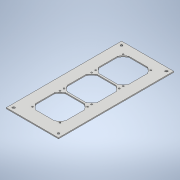
# Autodesk Inventor part: front_panel2
Saved by Autodesk Inventor 2022 (Build 260153000, 153)
## iProperties
Created: 2021-05-14
Part Number: front_panel2
Material: Generic
Document SubType Name: Modeling
Designer: gisen
Density: 1 g/cm^3
Appearance: Default
Author: gisen
Autodesk Inventor part; units mm, degrees
ref_plane "YZ Plane" through (0, 0, 0) normal (1, 0, 0) x (0, 1, 0)
ref_plane "XZ Plane" through (0, 0, 0) normal (0, 1, 0) x (-1, 0, 0)
ref_plane "XY Plane" through (0, 0, 0) normal (0, 0, 1) x (1, 0, 0)
sketch "Sketch1" plane through (0, 0, 0) normal (0, 0, 1) x (1, 0, 0)
  line L0 (-28.4765, -2.55) -> (28.4765, -2.55)
  arc A0 (44.7, -18.7735) -> (28.4765, -2.55) centre (0, -47.25) ccw
  line L1 (44.7, -18.7735) -> (44.7, -75.7265)
  arc A1 (28.4765, -91.95) -> (44.7, -75.7265) centre (0, -47.25) ccw
  line L2 (28.4765, -91.95) -> (-28.4765, -91.95)
  arc A2 (-44.7, -75.7265) -> (-28.4765, -91.95) centre (0, -47.25) ccw
  line L3 (-44.7, -75.7265) -> (-44.7, -18.7735)
  arc A3 (-28.4765, -2.55) -> (-44.7, -18.7735) centre (0, -47.25) ccw
  line L4 (-28.4765, 91.95) -> (28.4765, 91.95)
  arc A4 (44.7, 75.7265) -> (28.4765, 91.95) centre (0, 47.25) ccw
  line L5 (44.7, 75.7265) -> (44.7, 18.7735)
  arc A5 (28.4765, 2.55) -> (44.7, 18.7735) centre (0, 47.25) ccw
  line L6 (28.4765, 2.55) -> (-28.4765, 2.55)
  arc A6 (-44.7, 18.7735) -> (-28.4765, 2.55) centre (0, 47.25) ccw
  line L7 (-44.7, 18.7735) -> (-44.7, 75.7265)
  arc A7 (-28.4765, 91.95) -> (-44.7, 75.7265) centre (0, 47.25) ccw
  line L8 (-28.4765, 186.45) -> (28.4765, 186.45)
  arc A8 (44.7, 170.2265) -> (28.4765, 186.45) centre (0, 141.75) ccw
  line L9 (44.7, 170.2265) -> (44.7, 113.2735)
  arc A9 (28.4765, 97.05) -> (44.7, 113.2735) centre (0, 141.75) ccw
  line L10 (28.4765, 97.05) -> (-28.4765, 97.05)
  arc A10 (-44.7, 113.2735) -> (-28.4765, 97.05) centre (0, 141.75) ccw
  line L11 (-44.7, 113.2735) -> (-44.7, 170.2265)
  arc A11 (-28.4765, 186.45) -> (-44.7, 170.2265) centre (0, 141.75) ccw
  circle A12 centre (-41.25, -88.5) radius 2.25
  circle A13 centre (41.25, -88.5) radius 2.25
  circle A14 centre (41.25, -6) radius 2.25
  circle A15 centre (-41.25, -6) radius 2.25
  circle A16 centre (-41.25, 6) radius 2.25
  circle A17 centre (41.25, 6) radius 2.25
  circle A18 centre (41.25, 88.5) radius 2.25
  circle A19 centre (-41.25, 88.5) radius 2.25
  circle A20 centre (41.25, 183) radius 2.25
  circle A21 centre (41.25, 100.5) radius 2.25
  circle A22 centre (-41.25, 100.5) radius 2.25
  circle A23 centre (-41.25, 183) radius 2.25
  arc A24 (15.0245, 209.46) -> (15.0245, 194.54) centre (17.5, 202) ccw
  line L12 (15.0245, 209.46) -> (19.9755, 209.46)
  arc A25 (19.9755, 194.54) -> (19.9755, 209.46) centre (17.5, 202) ccw
  line L13 (19.9755, 194.54) -> (15.0245, 194.54)
  arc A26 (-15.0245, 194.54) -> (-15.0245, 209.46) centre (-17.5, 202) ccw
  line L14 (-15.0245, 194.54) -> (-19.9755, 194.54)
  arc A27 (-19.9755, 209.46) -> (-19.9755, 194.54) centre (-17.5, 202) ccw
  line L15 (-19.9755, 209.46) -> (-15.0245, 209.46)
  line L16 (-54.7, 214.7) -> (54.7, 214.7)
  line L17 (54.7, -129.8) -> (-54.7, -129.8)
  line L18 (-78, -129.8) -> (78, -129.8)
  line L19 (-78, -129.8) -> (-78, 214.7)
  arc A28 (-64.7298, -120.3577) -> (-68.5577, -116.5298) centre (-66.3, -118.1) ccw
  arc A29 (-70.1472, -118.8153) -> (-67.0153, -121.9472) centre (-68.3, -120.1) ccw
  line L20 (-67.0153, -121.9472) -> (-64.7298, -120.3577)
  line L21 (-70.1472, -118.8153) -> (-68.5577, -116.5298)
  arc A30 (68.5577, -116.5298) -> (64.7298, -120.3577) centre (66.3, -118.1) ccw
  arc A31 (67.0153, -121.9472) -> (70.1472, -118.8153) centre (68.3, -120.1) ccw
  line L22 (67.0153, -121.9472) -> (64.7298, -120.3577)
  line L23 (70.1472, -118.8153) -> (68.5577, -116.5298)
  line L24 (78, -129.8) -> (78, 214.7)
  arc A32 (-68.5577, 201.4298) -> (-64.7298, 205.2577) centre (-66.3, 203) ccw
  arc A33 (-67.0153, 206.8472) -> (-70.1472, 203.7153) centre (-68.3, 205) ccw
  line L25 (-67.0153, 206.8472) -> (-64.7298, 205.2577)
  line L26 (-70.1472, 203.7153) -> (-68.5577, 201.4298)
  line L27 (70.1472, 203.7153) -> (68.5577, 201.4298)
  arc A34 (64.7298, 205.2577) -> (68.5577, 201.4298) centre (66.3, 203) ccw
  line L28 (67.0153, 206.8472) -> (64.7298, 205.2577)
  arc A35 (70.1472, 203.7153) -> (67.0153, 206.8472) centre (68.3, 205) ccw
  line L29 (-78, 214.7) -> (78, 214.7)
  point P0 (-54.7, -129.8)
  point P1 (54.7, -129.8)
  point P2 (0, 205.2577)
  dimension "d197" = 156
  dimension "d199" = 344.5
  dimension "d221" = 344.5
  dimension "d224" = 9.7
  dimension "d225" = 9.7
  dimension "d228" = 11.7
  dimension "d229" = 11.7
  dimension "d232" = 5.5
  dimension "d233" = 4.5
  constraints: 60 end point, 48 point on circle, 36 centre point, 8 coincident, 4 tangent, 2 point on line, 2 vertical, 1 collinear, 1 horizontal
  measures "d197" distance of L18.start L18.end
  measures "d199" distance between parallel lines of L18 L16
  measures "d221" distance between parallel lines of L16 L17
  measures "d224" distance from line of L18 point (-68.3, -120.1)
  measures "d225" distance from line of L19 point (-68.3, -120.1)
  measures "d228" distance from line of L18 point (-66.3, -118.1)
  measures "d229" distance from line of point (-66.3, -118.1) L19
  measures "d232" diameter of A28
  measures "d233" diameter of A29
extrude "Extrusion1" add sketch "Sketch1" along normal blind 3
sketch "Sketch2" plane through (0, 0, 3) normal (0, 0, 1) x (1, 0, 0)
  line L0 (28.4765, 97.05) -> (-28.4765, 97.05) projected
  arc A0 (-44.7, 113.2735) -> (-28.4765, 97.05) centre (0, 141.75) ccw projected
  line L1 (-44.7, 113.2735) -> (-44.7, 170.2265) projected
  arc A1 (-28.4765, 186.45) -> (-44.7, 170.2265) centre (0, 141.75) ccw projected
  line L2 (-28.4765, 186.45) -> (28.4765, 186.45) projected
  arc A2 (44.7, 170.2265) -> (28.4765, 186.45) centre (0, 141.75) ccw projected
  line L3 (44.7, 170.2265) -> (44.7, 113.2735) projected
  arc A3 (28.4765, 97.05) -> (44.7, 113.2735) centre (0, 141.75) ccw projected
  line L4 (44.7, 75.7265) -> (44.7, 18.7735) projected
  arc A4 (28.4765, 2.55) -> (44.7, 18.7735) centre (0, 47.25) ccw projected
  line L5 (28.4765, 2.55) -> (-28.4765, 2.55) projected
  arc A5 (-44.7, 18.7735) -> (-28.4765, 2.55) centre (0, 47.25) ccw projected
  line L6 (-44.7, 18.7735) -> (-44.7, 75.7265) projected
  arc A6 (-28.4765, 91.95) -> (-44.7, 75.7265) centre (0, 47.25) ccw projected
  line L7 (-28.4765, 91.95) -> (28.4765, 91.95) projected
  arc A7 (44.7, 75.7265) -> (28.4765, 91.95) centre (0, 47.25) ccw projected
  arc A8 (28.4765, -91.95) -> (44.7, -75.7265) centre (0, -47.25) ccw projected
  line L8 (28.4765, -91.95) -> (-28.4765, -91.95) projected
  arc A9 (-44.7, -75.7265) -> (-28.4765, -91.95) centre (0, -47.25) ccw projected
  line L9 (-44.7, -75.7265) -> (-44.7, -18.7735) projected
  arc A10 (-28.4765, -2.55) -> (-44.7, -18.7735) centre (0, -47.25) ccw projected
  line L10 (-28.4765, -2.55) -> (28.4765, -2.55) projected
  arc A11 (44.7, -18.7735) -> (28.4765, -2.55) centre (0, -47.25) ccw projected
  line L11 (44.7, -18.7735) -> (44.7, -75.7265) projected
  line L12 (-15.0245, 194.54) -> (-19.9755, 194.54) projected
  arc A12 (-19.9755, 209.46) -> (-19.9755, 194.54) centre (-17.5, 202) ccw projected
  line L13 (-19.9755, 209.46) -> (-15.0245, 209.46) projected
  arc A13 (-15.0245, 194.54) -> (-15.0245, 209.46) centre (-17.5, 202) ccw projected
  line L14 (15.0245, 209.46) -> (19.9755, 209.46) projected
  arc A14 (19.9755, 194.54) -> (19.9755, 209.46) centre (17.5, 202) ccw projected
  line L15 (19.9755, 194.54) -> (15.0245, 194.54) projected
  arc A15 (15.0245, 209.46) -> (15.0245, 194.54) centre (17.5, 202) ccw projected
  arc A16 (64.7298, 205.2577) -> (68.5577, 201.4298) centre (66.3, 203) ccw projected
  line L16 (64.7298, 205.2577) -> (67.0153, 206.8472) projected
  arc A17 (70.1472, 203.7153) -> (67.0153, 206.8472) centre (68.3, 205) ccw projected
  line L17 (70.1472, 203.7153) -> (68.5577, 201.4298) projected
  arc A18 (-67.0153, 206.8472) -> (-70.1472, 203.7153) centre (-68.3, 205) ccw projected
  line L18 (-67.0153, 206.8472) -> (-64.7298, 205.2577) projected
  arc A19 (-68.5577, 201.4298) -> (-64.7298, 205.2577) centre (-66.3, 203) ccw projected
  line L19 (-68.5577, 201.4298) -> (-70.1472, 203.7153) projected
  arc A20 (67.0153, -121.9472) -> (70.1472, -118.8153) centre (68.3, -120.1) ccw projected
  line L20 (67.0153, -121.9472) -> (64.7298, -120.3577) projected
  arc A21 (68.5577, -116.5298) -> (64.7298, -120.3577) centre (66.3, -118.1) ccw projected
  line L21 (68.5577, -116.5298) -> (70.1472, -118.8153) projected
  arc A22 (-64.7298, -120.3577) -> (-68.5577, -116.5298) centre (-66.3, -118.1) ccw projected
  line L22 (-64.7298, -120.3577) -> (-67.0153, -121.9472) projected
  arc A23 (-70.1472, -118.8153) -> (-67.0153, -121.9472) centre (-68.3, -120.1) ccw projected
  line L23 (-70.1472, -118.8153) -> (-68.5577, -116.5298) projected
  circle A24 centre (41.25, 6) radius 2.25 projected
  circle A25 centre (41.25, 100.5) radius 2.25 projected
  circle A26 centre (41.25, 88.5) radius 2.25 projected
  circle A27 centre (-41.25, 100.5) radius 2.25 projected
  circle A28 centre (-41.25, 88.5) radius 2.25 projected
  circle A29 centre (-41.25, 6) radius 2.25 projected
  circle A30 centre (-41.25, -6) radius 2.25 projected
  circle A31 centre (41.25, -6) radius 2.25 projected
  circle A32 centre (41.25, 183) radius 2.25 projected
  circle A33 centre (-41.25, 183) radius 2.25 projected
  circle A34 centre (41.25, -88.5) radius 2.25 projected
  circle A35 centre (-41.25, -88.5) radius 2.25 projected
  line L24 (-78, -129.8) -> (78, -129.8) projected
  line L25 (78, -129.8) -> (78, 214.7) projected
  line L26 (78, 214.7) -> (-78, 214.7) projected
  line L27 (-78, 214.7) -> (-78, -129.8) projected
  point P0 (0, 0)
extrude "Extrusion2" add sketch "Sketch2" against normal up to surface (3 mm away) contours L12 A12 L13 A13 | L14 A14 L15 A15
equation "\"d221\" = d199"
equation "\"d224\" = d222"
equation "\"d225\" = d223"
equation "\"d229\" = d228"
equation "\"d222\" = 9.7"
equation "\"d223\" = 9.7"
body "Solid1"
